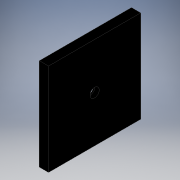
# Autodesk Inventor part: Robotunits CAP_4040_1
Saved by Autodesk Inventor 2019 (Build 230136000, 136)
## iProperties
Created: 2023-08-22
Part Number: Robotunits CAP_4040_1
Material: ABS PlastiK
Catalog Web Link: www.cadenas.de
Description: CAP_1-End Cap
Vendor: ROBOTUNITS
Document SubType Name: Modeling
Designer: psAdmin
Manufacturer: ROBOTUNITS
Mass: 6.69317 g
Surface Area: 38.5551 cm^2
Volume: 6.31431 cm^3
Density: 1.06 g/cm^3
Appearance: Generic
Category: PARTsolutions
Company: ROBOTUNITS
Title: Robotunits CAP_4040_1
Author: Cadenas PARTsolutions
Comments: End Cap
PSOL_IDENT_0: {$CADENAS_DATA/23d-libs/robotunits/pool_bauteile/cap.prj},181 {VTYP=3D},{NB=Robotunits CAP_4040_1},{
PSOL_IDENT_1: LINA=Robotunits CAP_4040_1},{NN=CAP_1},{DATE=24.04.2023 05:54:15},{GEOMDATE=22.02.2023 09:25:00},{VE
PSOL_IDENT_2: RSION=},{LINEID=10},{WBVAR=},{WBNUMERIC=}  {NB=Robotunits CAP_4040_1},{LINA=Robotunits CAP_4040_1},{
PSOL_IDENT_3: KT=DUMMY},{ARTIKEL=CAP_4040},{L=40},{B=40},{H=4},{GEW=0.005},{INFO=INFO},{V=1.000}
NB: Robotunits CAP_4040_1
NN: CAP_1
NT: End Cap
NBSYN: Robotunits $ARTIKEL._1
LINA: Robotunits CAP_4040_1
CATALOG: Robotunits
ARTIKEL: CAP_4040
L: 40
B: 40
H: 4
GEW: 0.005
INFO: INFO
SUPPLIER: ROBOTUNITS
ARTICLENO: Robotunits CAP_4040_1
BOMINFO: Robotunits CAP_4040_1
CREATOR: CADENAS GmbH
Autodesk Inventor part; units mm, degrees
ref_plane "YZ Plane" through (0, 0, 0) normal (1, 0, 0) x (0, 1, 0)
ref_plane "XZ Plane" through (0, 0, 0) normal (0, 1, 0) x (-1, 0, 0)
ref_plane "XY Plane" through (0, 0, 0) normal (0, 0, 1) x (1, 0, 0)
sketch "Skizze_1" plane through (0, 0, 0) normal (1, 0, 0) x (0, 0, -1)
  line L0 (-20, 20) -> (-20, -20)
  line L1 (-20, -20) -> (20, -20)
  line L2 (20, -20) -> (20, 20)
  line L3 (20, 20) -> (-20, 20)
  constraints: 8 end point
extrude "Extrusion1" add sketch "Skizze_1" along normal blind 4
sketch "Sketch2" plane through (0, 0, 0) normal (-1, 0, 0) x (0, 0, 1)
  point P0 (0, 0)
hole "Hole1" at (0, 0, 0) direction (1, 0, 0) diameter 4 depth 4 countersink diameter 8.1 countersink angle 90
ref_plane "CS_ANBAU_CAP_XY" through (0, 0, 0) normal (0, 1, 0) x (1, 0, 0)
ref_plane "CS_ANBAU_CAP_YZ" through (0, 0, 0) normal (1, 0, 0) x (0, 0, -1)
ref_plane "CS_ANBAU_CAP_ZX" through (0, 0, 0) normal (0, 0, -1) x (0, 1, 0)
ref_plane "CS_ANBAU_CAP_90_XY" through (0, 0, 0) normal (0, 0, 1) x (1, 0, 0)
ref_plane "CS_ANBAU_CAP_90_YZ" through (0, 0, 0) normal (1, 0, 0) x (0, 1, 0)
ref_plane "CS_ANBAU_CAP_90_ZX" through (0, 0, 0) normal (0, 1, 0) x (0, 0, 1)
ref_plane "IB_1_XY" through (0, 0, 0) normal (1, 0, 0) x (0, 0, -1)
ref_plane "IB_1_YZ" through (0, 0, 0) normal (0, 0, -1) x (0, 1, 0)
ref_plane "IB_1_ZX" through (0, 0, 0) normal (0, 1, 0) x (1, 0, 0)
ref_plane "IB_10_XY" through (0, -14, 10) normal (1, 0, 0) x (0, 0, -1)
ref_plane "IB_10_YZ" through (0, -14, 10) normal (0, 0, -1) x (0, 1, 0)
ref_plane "IB_10_ZX" through (0, -14, 10) normal (0, 1, 0) x (1, 0, 0)
ref_plane "IB_11_XY" through (0, 14, 10) normal (1, 0, 0) x (0, 0, -1)
ref_plane "IB_11_YZ" through (0, 14, 10) normal (0, 0, -1) x (0, 1, 0)
ref_plane "IB_11_ZX" through (0, 14, 10) normal (0, 1, 0) x (1, 0, 0)
ref_plane "IB_12_XY" through (0, 0, 0) normal (1, 0, 0) x (0, 0, -1)
ref_plane "IB_12_YZ" through (0, 0, 0) normal (0, 0, -1) x (0, 1, 0)
ref_plane "IB_12_ZX" through (0, 0, 0) normal (0, 1, 0) x (1, 0, 0)
ref_plane "IB_2_XY" through (0, 0, -10) normal (1, 0, 0) x (0, 0, -1)
ref_plane "IB_2_YZ" through (0, 0, -10) normal (0, 0, -1) x (0, 1, 0)
ref_plane "IB_2_ZX" through (0, 0, -10) normal (0, 1, 0) x (1, 0, 0)
ref_plane "IB_3_XY" through (0, 0, 10) normal (1, 0, 0) x (0, 0, -1)
ref_plane "IB_3_YZ" through (0, 0, 10) normal (0, 0, -1) x (0, 1, 0)
ref_plane "IB_3_ZX" through (0, 0, 10) normal (0, 1, 0) x (1, 0, 0)
ref_plane "IB_4_XY" through (0, 13.5, -13.5) normal (1, 0, 0) x (0, 0, -1)
ref_plane "IB_4_YZ" through (0, 13.5, -13.5) normal (0, 0, -1) x (0, 1, 0)
ref_plane "IB_4_ZX" through (0, 13.5, -13.5) normal (0, 1, 0) x (1, 0, 0)
ref_plane "IB_5_XY" through (0, 13.5, 13.5) normal (1, 0, 0) x (0, 0, -1)
ref_plane "IB_5_YZ" through (0, 13.5, 13.5) normal (0, 0, -1) x (0, 1, 0)
ref_plane "IB_5_ZX" through (0, 13.5, 13.5) normal (0, 1, 0) x (1, 0, 0)
ref_plane "IB_6_XY" through (0, 1.5, 6.5) normal (1, 0, 0) x (0, 0, -1)
ref_plane "IB_6_YZ" through (0, 1.5, 6.5) normal (0, 0, -1) x (0, 1, 0)
ref_plane "IB_6_ZX" through (0, 1.5, 6.5) normal (0, 1, 0) x (1, 0, 0)
ref_plane "IB_7_XY" through (0, 1.5, -6.5) normal (1, 0, 0) x (0, 0, -1)
ref_plane "IB_7_YZ" through (0, 1.5, -6.5) normal (0, 0, -1) x (0, 1, 0)
ref_plane "IB_7_ZX" through (0, 1.5, -6.5) normal (0, 1, 0) x (1, 0, 0)
ref_plane "IB_8_XY" through (0, -2, 14) normal (1, 0, 0) x (0, 0, -1)
ref_plane "IB_8_YZ" through (0, -2, 14) normal (0, 0, -1) x (0, 1, 0)
ref_plane "IB_8_ZX" through (0, -2, 14) normal (0, 1, 0) x (1, 0, 0)
ref_plane "IB_9_XY" through (0, -2, -14) normal (1, 0, 0) x (0, 0, -1)
ref_plane "IB_9_YZ" through (0, -2, -14) normal (0, 0, -1) x (0, 1, 0)
ref_plane "IB_9_ZX" through (0, -2, -14) normal (0, 1, 0) x (1, 0, 0)
body "Solid1"
